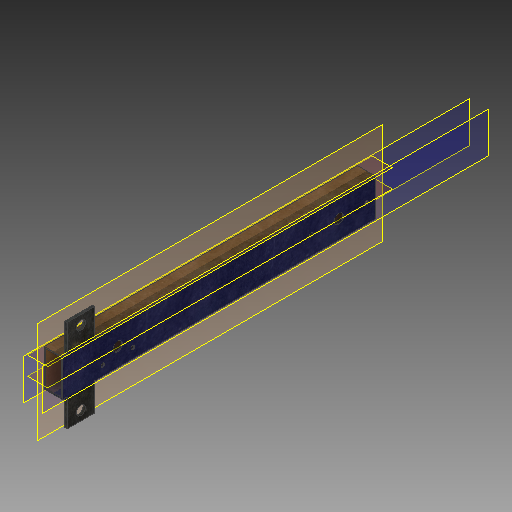
# Autodesk Inventor part: Steel 4130 1x2in. Tubing, t=.065in.,L=22in.
Saved by Autodesk Inventor 2019 (Build 230136000, 136)
## iProperties
Created: 2018-10-28
Part Number: Steel 4130 1x2in. Tubing, t=.065in.,L=22in.
Material: Steel
Document SubType Name: Modeling
Designer: Alex Barnett
Density: 7.85 g/cm^3
Appearance: Plate
Mass: 873.291 g
Surface Area: 1315.64 cm^2
Volume: 111.247 cm^3
Author: Alex Barnett
Autodesk Inventor part; units mm, degrees
ref_plane "XY Plane" through (0, 0, 0) normal (0, 0, 1) x (1, 0, 0)
sketch "Sketch1" plane through (0, 0, 0) normal (0, 0, 1) x (1, 0, 0)
  line L0 (-12.7, -25.4) -> (12.7, -25.4)
  line L1 (12.7, -25.4) -> (12.7, 25.4)
  line L2 (12.7, 25.4) -> (-12.7, 25.4)
  line L3 (-12.7, 25.4) -> (-12.7, -25.4)
  line L4 (-12.7, -25.4) -> (12.7, 25.4) construction
  line L5 (12.7, -25.4) -> (-12.7, 25.4) construction
  line L6 (-11.049, -23.749) -> (11.049, -23.749)
  line L7 (11.049, -23.749) -> (11.049, 23.749)
  line L8 (11.049, 23.749) -> (-11.049, 23.749)
  line L9 (-11.049, 23.749) -> (-11.049, -23.749)
  line L10 (-11.049, -23.749) -> (11.049, 23.749) construction
  line L11 (11.049, -23.749) -> (-11.049, 23.749) construction
  point P0 (0, 0)
  dimension "d0" = 25.4
  dimension "d1" = 50.8
  dimension "d4" = 22.098
  dimension "d5" = 47.498
  constraints: 24 end point, 4 midpoint, 4 parallel, 2 horizontal, 2 perpendicular
  measures "d0" distance of L2.end L1.end
  measures "d1" distance of L1.end L0.end
  measures "d4" distance of L8.end L7.end
  measures "d5" distance of L7.end L6.end
extrude "Extrusion2" add sketch "Sketch1" along normal mid plane 431.8
sketch "Sketch2" plane through (12.7, -25.4, 215.9) normal (1, 0, 0) x (0, 0, -1)
  line L0 (431.8, 50.8) -> (0, 50.8) projected
  line L1 (0, 0) -> (0, 50.8) projected
  line L2 (431.8, 0) -> (0, 0) projected
  line L3 (431.8, 50.8) -> (431.8, 0) projected
  point P0 (215.9, 25.4)
  point P1 (76.2, 25.4)
  dimension "d8" = 76.2
  dimension "d9" = 25.4
  measures "d8" distance from line of L1 point (76.2, 25.4)
  measures "d9" distance from line of L2 point (76.2, 25.4)
hole "Hole1" at (12.7, 0, 139.7) direction (-1, 0, 0) diameter 12.7 end through all
sketch "Sketch3" plane through (-12.7, -25.4, 215.9) normal (-1, 0, 0) x (0, 0, 1)
  circle A0 centre (-76.2, 25.4) radius 6.35 projected
  line L0 (0, 0) -> (-431.8, 0) projected
  line L1 (0, 50.8) -> (0, 0) projected
  line L2 (-431.8, 50.8) -> (0, 50.8) projected
  line L3 (-431.8, 0) -> (-431.8, 50.8) projected
  line L4 (-76.2, 25.4) -> (-34.0057, 1.0391) construction
  line L5 (-76.2, 25.4) -> (-27.4783, 25.4) construction
  line L6 (-76.2, 25.4) -> (-120.9567, -0.4403) construction
  line L7 (-76.2, 25.4) -> (-24.5194, 25.4) construction
  line L8 (-76.2, 25.4) -> (-76.2, 62.5709) construction
  circle A1 centre (-76.2, 25.4) radius 23.8125 construction
  point P0 (-215.9, 25.4)
  point P1 (-55.5778, 13.4937)
  point P2 (-96.8222, 13.4938)
  dimension "d17" = 30
  dimension "d18" = 150
  dimension "d19" = 47.625
  constraints: 10 end point, 2 equal length, 2 horizontal, 2 point on circle, 2 point on line, 1 centre point, 1 coincident, 1 vertical
  measures "d17" angle of L4 L5
  measures "d18" angle of L6 L7
  measures "d19" diameter of A1
hole "Hole2" at (-12.7, -11.9063, 160.3222) at (-12.7, -11.9062, 119.0778) direction (1, 0, 0) diameter 5.08 end through all
ref_plane "Work Plane1" through (-12.7, -25.4, 215.9) normal (-1, 0, 0) x (0, 0, 1)
ref_plane "Work Plane2" through (12.7, -25.4, 215.9) normal (-1, 0, 0) x (0, 0, 1)
sketch "Sketch4" plane through (-12.7, -25.4, 215.9) normal (-1, 0, 0) x (0, 0, 1)
  circle A0 centre (-55.5778, 13.4937) radius 2.54 projected
  circle A1 centre (-96.8222, 13.4938) radius 2.54 projected
  circle A2 centre (-76.2, 25.4) radius 6.35 projected
  line L0 (0, 0) -> (-431.8, 0) projected
  line L1 (0, 50.8) -> (0, 0) projected
  line L2 (-431.8, 50.8) -> (0, 50.8) projected
  line L3 (-431.8, 0) -> (-431.8, 50.8) projected
  point P0 (-215.9, 25.4)
  point P1 (-381, 25.4)
  dimension "d29" = 50.8
  dimension "d30" = 25.4
  measures "d29" distance from line of L3 point (-381, 25.4)
  measures "d30" distance from line of L2 point (-381, 25.4)
hole "Hole3" at (-12.7, 0, -165.1) direction (1, 0, 0) diameter 12.7 end through all
sketch "Sketch5" plane through (-12.7, -25.4, 215.9) normal (-1, 0, 0) x (0, 0, 1)
  circle A0 centre (-381, 25.4) radius 6.35 projected
  circle A1 centre (-55.5778, 13.4937) radius 2.54 projected
  circle A2 centre (-96.8222, 13.4938) radius 2.54 projected
  circle A3 centre (-76.2, 25.4) radius 6.35 projected
  line L0 (0, 0) -> (-431.8, 0) projected
  line L1 (0, 50.8) -> (0, 0) projected
  line L2 (-431.8, 50.8) -> (0, 50.8) projected
  line L3 (-431.8, 0) -> (-431.8, 50.8) projected
  point P0 (-215.9, 25.4)
  point P1 (-419.1, 25.4)
  point P2 (-342.9, 25.4)
  dimension "d38" = 38.1
  dimension "d39" = 76.2
  measures "d38" distance of A0.centre point (-419.1, 25.4)
  measures "d39" distance of point (-419.1, 25.4) point (-342.9, 25.4)
hole "Hole4" at (-12.7, 0, -203.2) at (-12.7, 0, -127) direction (1, 0, 0) diameter 5.08 end through all
ref_plane "Work Plane3" through (-12.7, 25.4, 215.9) normal (0, 1, 0) x (1, 0, 0)
sketch "Sketch6" plane through (12.7, -25.4, 215.9) normal (1, 0, 0) x (0, 0, -1)
  circle A0 centre (419.1, 25.4) radius 2.54 projected
  circle A1 centre (342.9, 25.4) radius 2.54 projected
  circle A2 centre (381, 25.4) radius 6.35 projected
  circle A3 centre (55.5778, 13.4937) radius 2.54 projected
  circle A4 centre (96.8222, 13.4938) radius 2.54 projected
  circle A5 centre (76.2, 25.4) radius 6.35 projected
  line L0 (431.8, 50.8) -> (0, 50.8) projected
  line L1 (0, 0) -> (0, 50.8) projected
  line L2 (431.8, 0) -> (0, 0) projected
  line L3 (431.8, 50.8) -> (431.8, 0) projected
  circle A6 centre (25.4, 76.2) radius 6.35
  line L4 (6.35, 50.8) -> (44.45, 50.8)
  line L5 (44.45, 50.8) -> (44.45, 88.9)
  line L6 (44.45, 88.9) -> (6.35, 88.9)
  line L7 (6.35, 88.9) -> (6.35, 50.8)
  point P0 (215.9, 25.4)
  dimension "d48" = 12.7
  dimension "d49" = 25.4
  dimension "d50" = 25.4
  dimension "d51" = 38.1
  dimension "d52" = 38.1
  dimension "d53" = 19.05
  constraints: 8 end point, 2 parallel, 1 centre point, 1 horizontal, 1 perpendicular, 1 point on line
  measures "d48" diameter of A6
  measures "d49" horizontal distance of L0.end A6.centre
  measures "d50" distance from line of L0 A6.centre
  measures "d51" distance of L6.end L5.end
  measures "d52" distance of L5.end L4.end
  measures "d53" distance from line of L5 A6.centre
extrude "Extrusion3" add sketch "Sketch6" against normal blind 3.175 contours L0 L7 L6 L5
mirror "Mirror2" about plane through (0, 0, 0) normal (0, 1, 0) of "Extrusion3"
body "Solid2"
